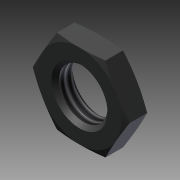
# Autodesk Inventor part: ZPT2_8_B_NUT
Saved by Autodesk Inventor 2011 SP1 (Build 150282100, 282)
## iProperties
Created: 2018-01-08
Part Number: ZPT2_8_B_NUT
Catalog Web Link: www.cadenas.de
Description: ZPT_2_8B_NUT-Vacuum Pad/Vertical Vacuum Entry With Buffer
Vendor: SMC
Document SubType Name: Modeling
Designer: psAdmin
Manufacturer: SMC
Mass: 0.252946 g
Surface Area: 3.44864 cm^2
Volume: 0.252946 cm^3
Density: 1 g/cm^3
Category: PARTsolutions
Company: SMC
Title: ZPT2_8_B_NUT
Author: Cadenas PARTsolutions
Comments: Vacuum Pad/Vertical Vacuum Entry With Buffer
PSOL_IDENT_0: {$CADENAS_DATA\23d-libs\smc_jp\vacuum_equipment\vacuum_pad\zp\zpt_b\zpt_2_8_b\parts\zpt_2_8_nut_b.pr
PSOL_IDENT_1: j},172 {VTYP=3D},{NB=ZPT2_8_B_NUT},{LINA=ZPT2_8_B_NUT},{NN=ZPT_2_8B_NUT},{DATE=12.07.2017 07:16:19},
PSOL_IDENT_2: {GEOMDATE=10.02.2011 07:48:00},{VERSION=},{LINEID=10},{LINESUBID=-1},{WBVAR=}  {NB=ZPT2_8_B_NUT},{LI
PSOL_IDENT_3: NA=ZPT2_8_B_NUT},{KT=DUMMY},{ORDER=ZPT2_8}
NN: ZPT_2_8B_NUT
NT: Vacuum Pad/Vertical Vacuum Entry With Buffer
NB: ZPT2_8_B_NUT
NBSYN: $ORDER._B_NUT
LINA: ZPT2_8_B_NUT
ORDER: ZPT2_8
SUPPLIER: SMC
ARTICLENO: ZPT2_8_B_NUT
BOMINFO: ZPT2_8_B_NUT
CREATOR: CADENAS GmbH
Autodesk Inventor part; units mm, degrees
sketch "Sketch_1" plane through (0, 0, 0) normal (0, 0, 1) x (1, 0, 0)
  line L0 (0, -1.5) -> (0, 1.5)
  line L1 (3.4585, 0.9585) -> (3.4585, -0.9585)
  line L2 (3.4585, -0.9585) -> (4, -1.5)
  line L3 (4, -1.5) -> (6, -1.5)
  line L4 (6, -1.5) -> (9.6, -0.5354)
  line L5 (9.6, -0.5354) -> (9.6, 0.5354)
  line L6 (9.6, 0.5354) -> (6, 1.5)
  line L7 (6, 1.5) -> (4, 1.5)
  line L8 (4, 1.5) -> (3.4585, 0.9585)
  constraints: 18 end point
revolve "Revolution1" add sketch "Sketch_1" angle 360 about axis through (0, -1.5, 0) along (0, -1, 0)
thread "Thread1" size "M8x1" class "6H" standard "ISO Metric profile" full length
sketch "Sketch_2" plane through (0, 0, 0) normal (0, 1, 0) x (-1, 0, 0)
  circle A0 centre (0, 0) radius 12
  line L0 (6.9282, 0) -> (3.4641, 6)
  line L1 (3.4641, 6) -> (-3.4641, 6)
  line L2 (-3.4641, 6) -> (-6.9282, 0)
  line L3 (-6.9282, 0) -> (-3.4641, -6)
  line L4 (-3.4641, -6) -> (3.4641, -6)
  line L5 (3.4641, -6) -> (6.9282, 0)
  constraints: 12 end point, 1 centre point
extrude "Extrusion1" cut sketch "Sketch_2" along normal mid plane 3
ref_plane "NUT_BUFFER_XY" through (0, 0, 0) normal (0, -1, 0) x (1, 0, 0)
ref_plane "NUT_BUFFER_YZ" through (0, 0, 0) normal (1, 0, 0) x (0, 0, 1)
ref_plane "NUT_BUFFER_ZX" through (0, 0, 0) normal (0, 0, 1) x (0, -1, 0)
body "Solid1"
